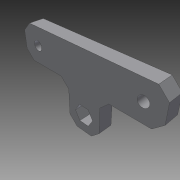
# Autodesk Inventor part: y_carriage_nut_holder_b
Saved by Autodesk Inventor 2014 (Build 180170000, 170)
## iProperties
Created: 2014-04-02
Part Number: y_carriage_nut_holder_b
Material: Plywood, Finish
Document SubType Name: Modeling
Designer: buben
Density: 0.552 g/cm^3
Appearance: Plywood - New
Author: buben
Autodesk Inventor part; units mm, degrees
ref_plane "YZ Plane" through (0, 0, 0) normal (1, 0, 0) x (0, 1, 0)
ref_plane "XZ Plane" through (0, 0, 0) normal (0, 1, 0) x (-1, 0, 0)
ref_plane "XY Plane" through (0, 0, 0) normal (0, 0, 1) x (1, 0, 0)
sketch "Sketch1" plane through (0, 0, 0) normal (0, 1, 0) x (-1, 0, 0)
  line L0 (0, -16) -> (0, 0)
  line L1 (0, 0) -> (-66, 0)
  line L2 (-66, 0) -> (-66, -16)
  line L3 (-66, -16) -> (-41, -16)
  line L4 (-41, -16) -> (-41, -36)
  line L5 (-41, -36) -> (-25, -36)
  line L6 (-25, -36) -> (-25, -16)
  line L7 (-25, -16) -> (0, -16)
  circle A0 centre (-8, -8) radius 2.25
  circle A1 centre (-58, -8) radius 2.25
  line L8 (-35.3094, -24) -> (-30.6906, -24)
  line L9 (-30.6906, -24) -> (-28.3812, -28)
  line L10 (-28.3812, -28) -> (-30.6906, -32)
  line L11 (-30.6906, -32) -> (-35.3094, -32)
  line L12 (-35.3094, -32) -> (-37.6188, -28)
  line L13 (-37.6188, -28) -> (-35.3094, -24)
  point P0 (0, -8)
  point P1 (-33, -28)
  point P2 (-33, -36)
  dimension "d0" = 16
  dimension "d1" = 4.5
  dimension "d2" = 50
  dimension "d3" = 8
  dimension "d4" = 8
  dimension "d5" = 16
  dimension "d6" = 36
  dimension "d7" = 8
  dimension "d8" = 20
  constraints: 28 end point, 6 parallel, 2 centre point, 2 collinear, 2 horizontal alignment, 2 midpoint, 1 equal radius, 1 horizontal, 1 perpendicular, 1 vertical, 1 vertical alignment, 13 other
  measures "d0" distance of L0.start L0.end
  measures "d1" diameter of A0
  measures "d2" distance of A1.centre A0.centre
  measures "d3" distance from line of L0 A0.centre
  measures "d4" distance from line of L2 A1.centre
  measures "d5" distance of L4.end L5.end
  measures "d6" distance between parallel lines of L1 L5
  measures "d7" distance between parallel lines of L8 L11
  measures "d8" vertical distance of point (-33, -28) A0.centre
extrude "Extrusion1" add sketch "Sketch1" along normal blind 6.5
chamfer "Chamfer1" distance 4 angle 45 8 edges at (66, 3.25, 0) (66, 3.25, -16) (0, 3.25, 0) (0, 3.25, -16) (25, 3.25, -16) (25, 3.25, -36) (41, 3.25, -36) (41, 3.25, -16)
equation "\"d3\" = 0.5 * d0"
equation "\"d4\" = d3"
body "Solid1"
